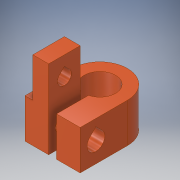
# Autodesk Inventor part: Piston Flag holder
Saved by Autodesk Inventor 2018.1 (Build 221171000, 171)
## iProperties
Created: 2013-10-19
Part Number: Piston Flag holder
Material: ABS Plastic
Document SubType Name: Modeling
Designer: Gabriel Smolnycki
Mass: 1.97286 g
Surface Area: 17.1051 cm^2
Volume: 1.86119 cm^3
Density: 1.06 g/cm^3
Appearance: Smooth - Light Orange
Author: Gabriel Smolnycki
Sending System: SolidWorks 2017
Last Author: Gabriel Smolnycki
Last Saved: 2017-09-14
Autodesk Inventor part; units mm, degrees
ref_plane "YZ Plane" through (0, 0, 0) normal (1, 0, 0) x (0, 1, 0)
ref_plane "XZ Plane" through (0, 0, 0) normal (0, 1, 0) x (-1, 0, 0)
ref_plane "XY Plane" through (0, 0, 0) normal (0, 0, 1) x (1, 0, 0)
sketch "Sketch1" plane through (0, 0, 0) normal (0, 1, 0) x (-1, 0, 0)
  line L0 (7, 0) -> (7, 12)
  arc A0 (-7, 0) -> (7, 0) centre (0, 0) ccw
  line L1 (-7, 12) -> (-7, 0)
  line L2 (-1, 3.873) -> (-1, 12)
  arc A1 (-1, 3.873) -> (1, 3.873) centre (0, 0) ccw
  line L3 (-1, 12) -> (-7, 12)
  line L4 (1, 12) -> (1, 3.873)
  line L5 (7, 12) -> (1, 12)
  constraints: 12 end point, 4 point on circle, 4 vertical, 3 equal length, 2 centre point, 2 horizontal, 1 collinear
extrude "Extrusion5" add sketch "Sketch1" along normal blind 20
sketch "Sketch2" plane through (0, 20, 0) normal (0, 1, 0) x (1, 0, 0)
  line L0 (-5, -4) -> (-1, -4)
  arc A0 (7, 0) -> (-7, 0) centre (0, 0) ccw
  line L1 (1, -12) -> (1, -3.873)
  line L2 (-5, -12) -> (-7, -12)
  line L3 (7, -12) -> (7, 0)
  arc A1 (1, -3.873) -> (-1, -3.873) centre (0, 0) ccw
  line L4 (-1, -3.873) -> (-1, -4)
  line L5 (-7, 0) -> (-7, -12)
  line L6 (1, -12) -> (7, -12)
  line L7 (-5, -4) -> (-5, -12)
  constraints: 16 end point, 5 vertical, 4 point on circle, 3 horizontal, 2 centre point, 1 collinear, 1 parallel
extrude "Extrusion4" cut sketch "Sketch2" against normal blind 10
sketch "Sketch3" plane through (-7, 0, 0) normal (-1, 0, 0) x (0, 0, 1)
  arc A0 (6.409, 6.591) -> (9.591, 6.591) centre (8, 5) ccw
  line L0 (8, 8.182) -> (6.409, 6.591)
  line L1 (9.591, 6.591) -> (8, 8.182)
  constraints: 4 end point, 2 perpendicular, 2 point on circle, 1 centre point
extrude "Extrusion3" cut sketch "Sketch3" against normal blind 6
sketch "Sketch4" plane through (7, 0, 12) normal (1, 0, 0) x (0, 0, -1)
  arc A0 (2.409, 6.591) -> (5.591, 6.591) centre (4, 5) ccw
  line L0 (2.409, 6.591) -> (4, 8.182)
  line L1 (4, 8.182) -> (5.591, 6.591)
  constraints: 4 end point, 2 perpendicular, 2 point on circle, 1 centre point
extrude "Extrusion2" cut sketch "Sketch4" against normal blind 6 draft 0
sketch "Sketch5" plane through (-5, 20, 4) normal (-1, 0, 0) x (0, 0, 1)
  line L0 (5.2374, -3.7626) -> (4, -2.5251)
  arc A0 (2.7626, -3.7626) -> (5.2374, -3.7626) centre (4, -5) ccw
  line L1 (4, -2.5251) -> (2.7626, -3.7626)
  constraints: 4 end point, 2 perpendicular, 2 point on circle, 1 centre point
extrude "Extrusion1" cut sketch "Sketch5" against normal blind 4
body "Solid3"
